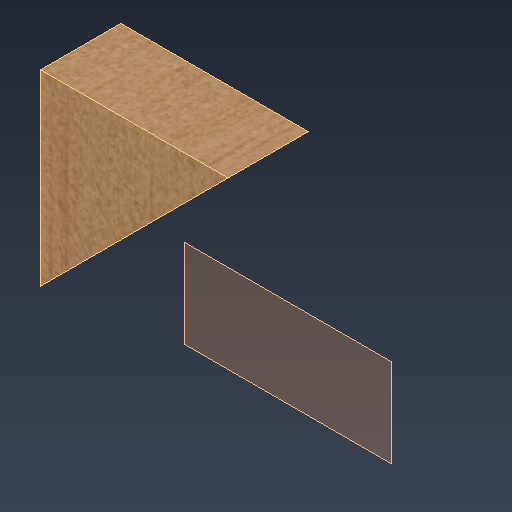
# Autodesk Inventor part: AesteticTriangle
Saved by Autodesk Inventor 2021 (Build 250183000, 183)
## iProperties
Created: 2017-09-10
Part Number: AesteticTriangle
Material: Wood
Document SubType Name: Modeling
Designer: jjsch
Density: 0.570257 g/cm^3
Appearance: Yellow Pine - Solid Natural Low Gloss
Mass: 85.8557 g
Surface Area: 194.675 cm^2
Volume: 150.556 cm^3
Author: jjsch
Autodesk Inventor part; units mm, degrees
ref_plane "YZ Plane" through (0, 0, 0) normal (1, 0, 0) x (0, 1, 0)
ref_plane "XZ Plane" through (0, 0, 0) normal (0, 1, 0) x (-1, 0, 0)
ref_plane "XY Plane" through (0, 0, 0) normal (0, 0, 1) x (1, 0, 0)
ref_plane "Work Plane1" through (72.936, -76.7222, 0) normal (0, 0, 1) x (1, 0, 0)
sketch "Sketch1" plane through (72.936, -76.7222, 0) normal (0, 0, 1) x (1, 0, 0)
  line L0 (-72.936, 76.7222) -> (15.964, 76.7222)
  line L1 (15.964, 76.7222) -> (-72.936, -12.1778)
  line L2 (-72.936, -12.1778) -> (-72.936, 76.7222)
  dimension "d0" = 88.9
  dimension "d1" = 45
  constraints: 6 end point, 1 horizontal, 1 perpendicular, 1 point on line
  measures "d0" distance of L0.start L0.end
  measures "d1" angle of L0 L1
extrude "Extrusion1" add sketch "Sketch1" against normal blind 38.1
body "Solid1"
